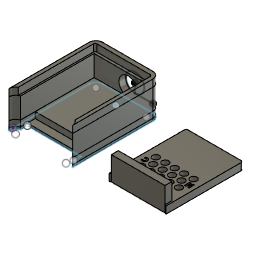
_Mini Radio Station-Simple Case.05f71377-dc7e-47c3-8c6b-2b0f3f518955 (Autodesk Fusion 360 design; units mm, degrees)
Autodesk Fusion 360 part; units mm, degrees
sketch "Sketch1" plane through (0, 0, 0) normal (0, 1, 0) x (1, 0, 0)
  line L0 (0, 0) -> (0, 1)
  line L1 (0, 1) -> (0, 28.94)
  line L2 (24.13, 28.94) -> (24.13, 1)
  line L3 (1.905, 3.54) -> (22.225, 3.54)
  line L4 (1.905, 1) -> (1.905, 3.54)
  line L5 (22.225, 1) -> (22.225, 3.54)
  line L6 (2.5, 31.44) -> (21.63, 31.44)
  arc A0 (2.5, 31.44) -> (0, 28.94) centre (2.5, 28.94) ccw
  arc A1 (24.13, 28.94) -> (21.63, 31.44) centre (21.63, 28.94) ccw
  line L7 (24.13, 1) -> (24.13, -1.5)
  line L8 (22.225, 1) -> (22.225, 0.89)
  line L9 (1.905, 1) -> (1.905, 0.9282)
  line L10 (0, 1) -> (0, -1.5)
  arc A2 (24.13, -1.5) -> (22.225, 0.9282) centre (21.63, -1.5) ccw
  arc A3 (1.905, 0.9282) -> (0, -1.5) centre (2.5, -1.5) ccw
  circle A4 centre (12.065, 26.96) radius 0.75
  dimension "d2" = 1
  dimension "d3" = 24.13
  dimension "d4" = 27.94
  dimension "d10" = 20.32
  dimension "d13" = 2.5
  dimension "d14" = 2.5
  dimension "d15" = 19.13
  dimension "d19" = 2.5
  dimension "d20" = 2.5
  dimension "d21" = 2.6118
  dimension "d22" = 2.54
  dimension "d109" = 1.5
  constraint coincident L0.start origin
  constraint vertical L0
  constraint perpendicular L3 L5
  constraint tangent L6 A1
  constraint tangent L10 A3
  constraint coincident L8 A2.end
  measures "d2" distance of L0.start L0.end
  measures "d3" distance of L0.end L2.end
  measures "d4" distance of L0.end L1.end
  measures "d10" distance of L4.start L5.start
  measures "d13" radius of A0
  measures "d14" radius of A1
  measures "d15" distance of L6.start L6.end
  measures "d19" radius of A2
  measures "d20" radius of A3
  measures "d21" distance of L3.start L9.end
  measures "d22" distance of L3.end L5.start
  measures "d109" diameter of A4
extrude "Extrude1" add sketch "Sketch1" along normal blind 0.8 contours L0 L1 L2 L3 L4 L5 L6 A0 A1 L7 L8 L9 L10 A2 A3 | A4 makes body 1
sketch "Sketch2" plane through (0, 0.8, 0) normal (0, 1, 0) x (-1, 0, 0)
  line L0 (-1.905, -0.9282) -> (-1.905, -3.54)
  line L1 (-1.905, -3.54) -> (-22.225, -3.54)
  line L2 (-22.225, -3.54) -> (-22.225, -0.9282)
  arc A0 (-24.13, 1.5) -> (-22.225, -0.9282) centre (-21.63, 1.5) ccw
  line L3 (-24.13, 1.5) -> (-24.13, -28.94)
  arc A1 (-24.13, -28.94) -> (-21.63, -31.44) centre (-21.63, -28.94) ccw
  line L4 (-21.63, -31.44) -> (-2.5, -31.44)
  arc A2 (-2.5, -31.44) -> (0, -28.94) centre (-2.5, -28.94) ccw
  line L5 (0, -28.94) -> (0, 1.5)
  arc A3 (-1.905, -0.9282) -> (0, 1.5) centre (-2.5, 1.5) ccw
  line L6 (-1.905, -3.54) -> (-1.905, -6.54)
  line L7 (-22.225, -3.54) -> (-22.225, -6.54)
  line L8 (-1.905, -6.54) -> (-22.225, -6.54)
  dimension "d27" = 3
  dimension "d28" = 3
  constraint coincident L0.end L1.start
  constraint perpendicular L1 L6
  constraint coincident L1.end L2.start
  constraint perpendicular L1 L7
  measures "d27" distance of L0.end L6.end
  measures "d28" distance of L1.end L7.end
extrude "Extrude2" add sketch "Sketch2" along normal blind 2.3 contours L0 L2 A0 L3 A1 L4 A2 L5 A3 L6 L7 L8 bodies 1
split "Split1" by plane through (0, 0.8, 0) normal (0, 1, 0) bodies 1 makes body 2 at (15.4517, 3.1, -21.4733)
sketch "Sketch4" plane through (0, 3.1, 0) normal (0, 1, 0) x (-1, 0, 0)
  line L0 (-1.905, -0.9282) -> (-1.905, -6.54)
  line L1 (-1.905, -6.54) -> (-22.225, -6.54)
  line L2 (-22.225, -6.54) -> (-22.225, -0.9282)
  arc A0 (-24.13, 1.5) -> (-22.225, -0.9282) centre (-21.63, 1.5) ccw
  line L3 (-24.13, 1.5) -> (-24.13, -28.94)
  arc A1 (-24.13, -28.94) -> (-21.63, -31.44) centre (-21.63, -28.94) ccw
  line L4 (-21.63, -31.44) -> (-2.5, -31.44)
  arc A2 (-2.5, -31.44) -> (0, -28.94) centre (-2.5, -28.94) ccw
  line L5 (0, -28.94) -> (0, 1.5)
  arc A3 (-1.905, -0.9282) -> (0, 1.5) centre (-2.5, 1.5) ccw
  line L6 (-1.905, -0.9282) -> (-1.905, -28.8682)
  line L7 (-1.905, -28.8682) -> (-22.225, -28.8682)
  line L8 (-22.225, -28.8682) -> (-22.225, -0.9282)
  dimension "d31" = 27.94
  dimension "d32" = 20.32
  constraint coincident L0.start A3.start
  constraint perpendicular L1 L6
  constraint perpendicular L6 L7
  constraint coincident L2.end A0.end
  measures "d31" distance of L0.start L6.end
  measures "d32" distance of L6.end L7.end
extrude "Extrude3" add sketch "Sketch4" along normal blind 1.6 contours L0 L2 A0 L3 A1 L4 A2 L5 A3 L6 L7 L8 bodies 2
split "Split2" by plane through (0, 3.1, 0) normal (0, 1, 0) bodies 2 makes body 3 at (15.2533, 4.7, -29.7254)
sketch "Sketch5" plane through (0, 4.7, 0) normal (0, 1, 0) x (-1, 0, 0)
  line L0 (-1.905, -0.9282) -> (-1.905, -28.8682)
  line L1 (-1.905, -28.8682) -> (-22.225, -28.8682)
  line L2 (-22.225, -28.8682) -> (-22.225, -0.9282)
  arc A0 (-24.13, 1.5) -> (-22.225, -0.9282) centre (-21.63, 1.5) ccw
  line L3 (-24.13, 1.5) -> (-24.13, -28.94)
  arc A1 (-24.13, -28.94) -> (-21.63, -31.44) centre (-21.63, -28.94) ccw
  line L4 (-21.63, -31.44) -> (-2.5, -31.44)
  arc A2 (-2.5, -31.44) -> (0, -28.94) centre (-2.5, -28.94) ccw
  line L5 (0, -28.94) -> (0, 1.5)
  arc A3 (-1.905, -0.9282) -> (0, 1.5) centre (-2.5, 1.5) ccw
  line L6 (-1.905, -3.54) -> (-22.225, -3.54)
  constraint horizontal L6
extrude "Extrude4" add sketch "Sketch5" along normal blind 6.3 contours L0 L1 L2 A0 L3 A1 L4 A2 L5 A3 bodies 3
sketch "Sketch6" plane through (0, 11, 0) normal (0, 1, 0) x (-1, 0, 0)
  line L0 (-1.905, -28.8682) -> (-22.225, -28.8682)
  line L1 (-22.225, -28.8682) -> (-22.225, -0.9282)
  arc A0 (-24.13, 1.5) -> (-22.225, -0.9282) centre (-21.63, 1.5) ccw
  line L2 (-24.13, 1.5) -> (-24.13, -28.94)
  arc A1 (-24.13, -28.94) -> (-21.63, -31.44) centre (-21.63, -28.94) ccw
  line L3 (-21.63, -31.44) -> (-2.5, -31.44)
  arc A2 (-2.5, -31.44) -> (0, -28.94) centre (-2.5, -28.94) ccw
  line L4 (0, -28.94) -> (0, 1.5)
  arc A3 (-1.905, -0.9282) -> (0, 1.5) centre (-2.5, 1.5) ccw
  line L5 (-1.905, -0.9282) -> (-1.905, -28.8682)
  line L6 (-1.305, -0.6959) -> (-1.305, -29.2432)
  line L7 (-22.825, -29.2432) -> (-22.825, -0.6959)
  line L8 (-1.93, -29.8682) -> (-22.2, -29.8682)
  arc A4 (-1.93, -29.8682) -> (-1.305, -29.2432) centre (-1.93, -29.2432) ccw
  arc A5 (-22.825, -29.2432) -> (-22.2, -29.8682) centre (-22.2, -29.2432) ccw
  dimension "d40" = 0.625
  dimension "d41" = 0.625
  constraint tangent L6 A4
  constraint tangent L8 A4
  constraint tangent L8 A5
  constraint tangent L7 A5
  constraint coincident A3 L6.start
  constraint coincident A0 L7.end
  measures "d40" radius of A4
  measures "d41" radius of A5
extrude "Extrude5" add sketch "Sketch6" along normal blind 2.7 contours A0 L2 A1 L3 A2 L4 A3 L6 L7 L8 A4 A5 bodies 3
split "Split3" by plane through (0, 11, 0) normal (0, 1, 0) bodies 3 makes body 4 at (15.2533, 13.7, -30.3921)
sketch "Sketch7" plane through (0, 4.7, 0) normal (0, 1, 0) x (-1, 0, 0)
  line L0 (-1.905, -3.54, 12) -> (-22.225, -3.54, 12)
  line L1 (-1.905, -3.54, 12) -> (-22.225, -3.54, 12)
  line L2 (-22.225, -3.54, 12) -> (-22.225, -0.928, 12)
  line L3 (-1.905, -3.54, 12) -> (-1.905, -0.928, 12)
  line L4 (-1.905, -0.928, 12) -> (-22.225, -0.928, 12)
  dimension "d44" = 2.612
  dimension "d45" = 2.612
extrude "Extrude6" add sketch "Sketch7" along normal blind 6 separate body contours L0 L1 L2 L3 L4 in plane through (0, 16.7, 0) normal (0, 1, 0) makes body 5
sketch "Sketch8" plane through (0, 22.7, 0) normal (0, 1, 0) x (-1, 0, 0)
  line L0 (-1.905, -3.54) -> (-1.905, -0.928)
  line L1 (-1.905, -0.928) -> (-22.225, -0.928)
  line L2 (-22.225, -0.928) -> (-22.225, -3.54)
  line L3 (-22.225, -3.54) -> (-1.905, -3.54)
  line L4 (-1.305, -0.6957) -> (-1.305, -29.243)
  line L5 (-22.825, -0.6957) -> (-22.825, -29.243)
  line L6 (-1.93, -29.868) -> (-22.2, -29.868)
  arc A0 (-1.93, -29.868) -> (-1.305, -29.243) centre (-1.93, -29.243) ccw
  arc A1 (-22.825, -29.243) -> (-22.2, -29.868) centre (-22.2, -29.243) ccw
  arc A2 (-22.825, -0.6957) -> (-22.225, -0.928) centre (-21.6299, 1.5001) ccw
  arc A3 (-1.905, -0.928) -> (-1.305, -0.6957) centre (-2.5, 1.5002) ccw
  line L7 (-1.905, -0.928) -> (-1.905, -6.928)
  line L8 (-1.905, -0.928) -> (-1.905, -6.928)
  circle A4 centre (-4.905, -9.228) radius 1.25
  circle A5 centre (-8.485, -9.228) radius 1.25
  circle A6 centre (-12.065, -9.228) radius 1.25
  circle A7 centre (-15.645, -9.228) radius 1.25
  circle A8 centre (-19.225, -9.228) radius 1.25
  circle A9 centre (-6.695, -12.018) radius 1.25
  circle A10 centre (-10.275, -12.018) radius 1.25
  circle A11 centre (-13.855, -12.018) radius 1.25
  circle A12 centre (-17.435, -12.018) radius 1.25
  circle A13 centre (-4.905, -14.808) radius 1.25
  circle A14 centre (-8.485, -14.808) radius 1.25
  circle A15 centre (-12.065, -14.808) radius 1.25
  circle A16 centre (-15.645, -14.808) radius 1.25
  circle A17 centre (-19.225, -14.808) radius 1.25
  line L9 (-2.815, -11.018) -> (-2.815, -13.018)
  line L10 (-2.815, -13.018) -> (-3.315, -13.018)
  line L11 (-2.815, -11.018) -> (-3.315, -11.018)
  line L12 (-3.315, -11.018) -> (-3.315, -12.518)
  line L13 (-4.065, -11.018) -> (-4.565, -11.018)
  line L14 (-4.565, -11.018) -> (-4.565, -13.018)
  line L15 (-4.565, -13.018) -> (-4.065, -13.018)
  line L16 (-3.315, -13.018) -> (-4.065, -11.518)
  line L17 (-3.315, -12.518) -> (-4.065, -11.018)
  line L18 (-4.065, -13.018) -> (-4.065, -11.518)
  line L19 (-20.9536, -11.6464) -> (-21.3071, -11.2929)
  line L20 (-20.9536, -12.3536) -> (-21.3071, -12.7071)
  arc A18 (-21.3071, -12.7071) -> (-21.3071, -11.2929) centre (-20.6, -12) ccw
  arc A19 (-20.9536, -12.3536) -> (-20.9536, -11.6464) centre (-20.6, -12) ccw
  line L21 (-1.905, -28.868) -> (-12.065, -28.868)
  circle A20 centre (-12.065, -26.963) radius 0.75
  dimension "d48" = 27.94
  dimension "d53" = 0.625
  dimension "d54" = 0.625
  dimension "d60" = 6
  dimension "d62" = 2.5
  dimension "d65" = -14.32
  dimension "d66" = 0
  dimension "d69" = 2.5
  dimension "d72" = -10.74
  dimension "d73" = 0
  dimension "d75" = 2.5
  dimension "d79" = -14.32
  dimension "d80" = 0
  dimension "d82" = 2
  dimension "d83" = 0.5
  dimension "d84" = 0.5
  dimension "d91" = 0.5
  dimension "d94" = 2
  dimension "d96" = 10.16
  dimension "d97" = 1.905
  dimension "d99" = 1.5
  constraint tangent L4 A0
  constraint tangent L6 A0
  constraint tangent L5 A1
  constraint tangent L6 A1
  constraint coincident L0.end L1.start
  constraint perpendicular L1 L7
  constraint parallel L7 L8
  constraint perpendicular L9 L10
  constraint perpendicular L9 L11
  constraint perpendicular L14 L15
  constraint parallel L16 L17
  constraint perpendicular L15 L18
  constraint concentric A18 A19
  measures "d48" distance of L0.end L21.start
  measures "d53" radius of A0
  measures "d54" radius of A1
  measures "d60" distance of L0.end L7.end
  measures "d62" diameter of A4
  measures "d69" diameter of A9
  measures "d75" diameter of A13
  measures "d82" distance of L9.start L9.end
  measures "d83" distance of L9.end L10.end
  measures "d84" distance of L9.start L11.end
  measures "d91" distance of L14.end L15.end
  measures "d94" diameter of A18
  measures "d96" distance of L21.start L21.end
  measures "d97" distance of L21.end A20.centre
  measures "d99" diameter of A20
extrude "Extrude7" add sketch "Sketch8" against normal blind 2.7 contours L0 L2 L3 L4 L5 L6 A0 A1 A2 A3 L7 L8 bodies 5
sketch "Sketch9" plane through (0, 0, -31.44) normal (0, 0, -1) x (-1, 0, 0)
  line L0 (-2.5, 11) -> (-21.63, 11)
  line L1 (-21.63, 11) -> (-21.63, 3.1)
  line L2 (-21.63, 3.1) -> (-2.5, 3.1)
  line L3 (-2.5, 3.1) -> (-2.5, 11)
  line L4 (-21.63, 3.1) -> (-14.835, 3.1)
  line L5 (-14.835, 3.1) -> (-14.835, 6.6)
  circle A0 centre (-14.835, 6.6) radius 3.5
  dimension "d102" = 6.795
  dimension "d118" = 3.5
  constraint coincident L1.end L2.start
  constraint perpendicular L1 L4
  constraint perpendicular L2 L5
  constraint coincident L5.end A0.centre
  constraint coincident L4.end A0
  measures "d102" distance of L1.end L4.end
  measures "d118" distance of L4.end L5.end
hole "Hole3" at (14.835, 6.35, -31.44) direction (0, 0, 1) diameter 6.5 depth 5 tip angle 118 bodies 3
delete_face "DeleteFace3" 2 faces at (12.1049, 8.1133, -30.5827) (15.1586, 9.5839, -30.5827) on bodies 3
hole "Hole4" at (14.835, 6.6, -31.44) direction (0, 0, 1) diameter 7 depth 5 tip angle 118 bodies 3
extrude "Extrude8" add 1 faces at (8.6783, 16.7, -2.6693) along direction (0, -1, 0) blind 3 on bodies 5 bodies 5
delete_face "DeleteFace4" 1 faces at (11.3602, 20.9, -27.2195) on bodies 5
move_body "Move3" bodies 5 to x (-1, 0, 0) y (0, -1, 0) z (0, 0, 1) at (59.61, 22.7, 0)
move_body "Move4" bodies 5 to x (1, 0, 0) y (0, 1, 0) z (0, 0, 1) at (-1, 0, 0)
hole "Hole1" [suppressed]
sketch "Sketch11" plane through (0, 3.1, 0) normal (0, 1, 0) x (-1, 0, 0)
  line L0 (-1.905, -6.54) -> (-22.225, -6.54)
  line L1 (-22.225, -6.54) -> (-22.225, -0.9282)
  arc A0 (-24.13, 1.5) -> (-22.225, -0.9282) centre (-21.63, 1.5) ccw
  line L2 (-24.13, 1.5) -> (-24.13, -28.94)
  arc A1 (-24.13, -28.94) -> (-21.63, -31.44) centre (-21.63, -28.94) ccw
  line L3 (-21.63, -31.44) -> (-2.5, -31.44)
  arc A2 (-2.5, -31.44) -> (0, -28.94) centre (-2.5, -28.94) ccw
  line L4 (0, -28.94) -> (0, 1.5)
  arc A3 (-1.905, -0.9282) -> (0, 1.5) centre (-2.5, 1.5) ccw
  line L5 (-1.905, -0.9282) -> (-1.905, -6.54)
delete_face "DeleteFace1" [suppressed]
move_body "Move1" [suppressed]
move_body "Move2" [suppressed]
hole "Hole2" [suppressed]
delete_face "DeleteFace2" [suppressed]
